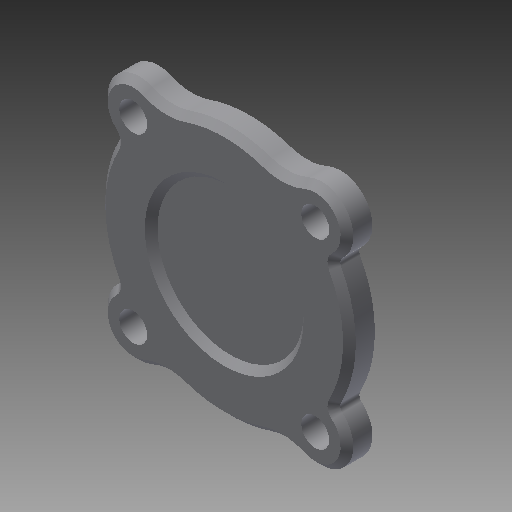
# Autodesk Inventor part: Crankshaft Cover
Saved by Autodesk Inventor 2017 (Build 210135000, 135)
## iProperties
Created: 2013-05-05
Part Number: Crankshaft Cover
Material: Generic
Document SubType Name: Modeling
Designer: John
Density: 1 g/cm^3
Appearance: Default
Author: John
Autodesk Inventor part; units mm, degrees
ref_plane "YZ Plane" through (0, 0, 0) normal (1, 0, 0) x (0, 1, 0)
ref_plane "XZ Plane" through (0, 0, 0) normal (0, 1, 0) x (-1, 0, 0)
ref_plane "XY Plane" through (0, 0, 0) normal (0, 0, 1) x (1, 0, 0)
sketch "Sketch1" plane through (0, 0, 0) normal (0, 0, 1) x (1, 0, 0)
  circle A0 centre (0, 0) radius 10.4775 projected
  circle A1 centre (9.0932, -9.0932) radius 0.9652 projected
  circle A2 centre (-9.0932, 9.0932) radius 0.9652 projected
  circle A3 centre (9.0932, 9.0932) radius 0.9652 projected
  circle A4 centre (-9.0932, -9.0932) radius 0.9652 projected
  arc A5 (11.1694, 6.6911) -> (7.7987, 11.9923) centre (9.0932, 9.0932) ccw projected
  arc A6 (4.0733, 11.8277) -> (7.7987, 11.9923) centre (5.7275, 16.6309) ccw projected
  arc A7 (4.0733, 11.8277) -> (-4.0733, 11.8277) centre (0, 0) ccw projected
  arc A8 (-7.7987, 11.9923) -> (-4.0733, 11.8277) centre (-5.7275, 16.6309) ccw projected
  arc A9 (-7.7987, 11.9923) -> (-11.1694, 6.6911) centre (-9.0932, 9.0932) ccw projected
  arc A10 (-11.025, 5.9107) -> (-11.1694, 6.6911) centre (-11.5847, 6.2107) ccw projected
  arc A11 (-11.025, 5.9107) -> (-11.025, -5.9107) centre (0, 0) ccw projected
  arc A12 (-11.1694, -6.6911) -> (-11.025, -5.9107) centre (-11.5847, -6.2107) ccw projected
  arc A13 (-11.1694, -6.6911) -> (-7.7987, -11.9923) centre (-9.0932, -9.0932) ccw projected
  arc A14 (-4.0733, -11.8277) -> (-7.7987, -11.9923) centre (-5.7275, -16.6309) ccw projected
  arc A15 (-4.0733, -11.8277) -> (4.0733, -11.8277) centre (0, 0) ccw projected
  arc A16 (7.7987, -11.9923) -> (4.0733, -11.8277) centre (5.7275, -16.6309) ccw projected
  arc A17 (7.7987, -11.9923) -> (11.1694, -6.6911) centre (9.0932, -9.0932) ccw projected
  arc A18 (11.025, -5.9107) -> (11.1694, -6.6911) centre (11.5847, -6.2107) ccw projected
  arc A19 (11.025, -5.9107) -> (11.025, 5.9107) centre (0, 0) ccw projected
  arc A20 (11.1694, 6.6911) -> (11.025, 5.9107) centre (11.5847, 6.2107) ccw projected
  point P0 (0, 0)
extrude "Extrusion1" add sketch "Sketch1" along normal blind 2.54 contours A0 | A1 | A2 | A3 | A4 | A20 A19 A18 A17 A16 A15 A14 A13 A12 A11 A10 A9 A8 A7 A6 A5
sketch "Sketch2" plane through (0, 0, 0) normal (0, 0, -1) x (-1, 0, 0)
  circle A0 centre (0, 0) radius 10.4775 projected
  circle A1 centre (0, 0) radius 10.3505
  dimension "d2" = 0.127
  constraints: 1 centre point, 1 coincident
  measures "d2" radial gap between concentric circles of A0 A1
extrude "Extrusion2" add sketch "Sketch2" along normal blind 0.635 contours A1
sketch "Sketch3" plane through (0, 0, -0.635) normal (0, 0, -1) x (-1, 0, 0)
  circle A0 centre (0, 0) radius 4.0005 projected
  circle A1 centre (0, 0) radius 4.0259
  circle A2 centre (0, 0) radius 6.5659
  dimension "d5" = 0.0254
  dimension "d6" = 2.54
  constraints: 2 centre point, 2 coincident
  measures "d5" radial gap between concentric circles of A0 A1
  measures "d6" radial gap between concentric circles of A2 A1
extrude "Extrusion3" add sketch "Sketch3" along normal blind 3.175 contours A2
chamfer "Chamfer1" distance 0.635 angle 45 1 edges at (6.5659, 0, -3.81)
chamfer "Chamfer4" distance 0.254 angle 45 1 edges at (10.3505, 0, -0.635)
sketch "Sketch4" plane through (0, 0, 2.54) normal (0, 0, 1) x (1, 0, 0)
  arc A0 (11.1694, 6.6911) -> (7.7987, 11.9923) centre (9.0932, 9.0932) ccw projected
  arc A1 (-7.7987, 11.9923) -> (-11.1694, 6.6911) centre (-9.0932, 9.0932) ccw projected
  arc A2 (-11.1694, -6.6911) -> (-7.7987, -11.9923) centre (-9.0932, -9.0932) ccw projected
  arc A3 (7.7987, -11.9923) -> (11.1694, -6.6911) centre (9.0932, -9.0932) ccw projected
hole "Hole1" at (9.0932, 9.0932, 2.54) at (-9.0932, 9.0932, 2.54) at (-9.0932, -9.0932, 2.54) at (9.0932, -9.0932, 2.54) direction (0, 0, -1) diameter 2.794 end through all clearance for "Flat Head Machine Screw (82)" size "#3" standard "Ansi Unified Screw Threads"
sketch "Sketch5" plane through (0, 0, 2.54) normal (0, 0, 1) x (1, 0, 0)
  arc A0 (11.025, -5.9107) -> (11.025, 5.9107) centre (0, 0) ccw projected
  circle A1 centre (0, 0) radius 7.9375
  dimension "d19" = 15.875
  constraints: 1 centre point, 1 coincident
  measures "d19" diameter of A1
extrude "Extrusion4" cut sketch "Sketch5" against normal blind 0.635
chamfer "Chamfer2" distance 0.635 angle 45 1 edges at (-7.9375, 0, 1.905)
chamfer "Chamfer3" distance 0.635 angle 45 16 edges at (12.5095, 0, 2.54) (10.9603, 6.3263, 2.54) (11.7724, 10.7968, 2.54) (5.9517, 11.5558, 2.54) (0, 12.5095, 2.54) (-5.9517, 11.5558, 2.54) (-11.7724, 10.7968, 2.54) (-10.9603, 6.3263, 2.54) (-12.5095, 0, 2.54) (-10.9603, -6.3263, 2.54) (-11.7724, -10.7968, 2.54) (-5.9517, -11.5558, 2.54) (0, -12.5095, 2.54) (5.9517, -11.5558, 2.54) (11.7724, -10.7968, 2.54) (10.9603, -6.3263, 2.54)
body "Solid1"
